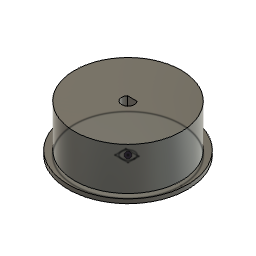
shaft v1 (Autodesk Fusion 360 design; units mm, degrees)
Autodesk Fusion 360 part; units mm, degrees
sketch "스케치1" plane through (0, 0, 0) normal (0, 1, 0) x (1, 0, 0)
  circle A0 centre (0, 0) radius 3
  line L0 (-3, 2) -> (3, 2)
  line L1 (3, 2) -> (3, -3)
  line L2 (3, -3) -> (-3, -3)
  line L3 (-3, -3) -> (-3, 2)
  circle A1 centre (0, 0) radius 25
  dimension "d1" = 6
  dimension "d2" = 5
  dimension "d3" = 50
  constraint coincident A0.centre A1.centre
  constraint horizontal L0
  constraint vertical L1
  constraint horizontal L2
  constraint vertical L3
  constraint tangent A0 L2
  constraint tangent A0 L1
  constraint tangent A0 L3
  measures "d1" diameter of A0
  measures "d2" distance of L0 L2
  measures "d3" diameter of A1
extrude "돌출1" add sketch "스케치1" along normal blind 22 contours A0 L1 L2 | A0 L0 L1 | A0 L0 | A0 L2 L3 | A0 L0 L3 | A1 picked at (-0.1397, 2.3235)
sketch "스케치2" plane through (0, 0, 0) normal (0, 1, 0) x (1, 0, 0)
  circle A0 centre (0, 0) radius 28
  dimension "d6" = 56
  constraint coincident A0.centre origin
  measures "d6" diameter of A0
extrude "돌출2" add sketch "스케치2" along normal blind 2
